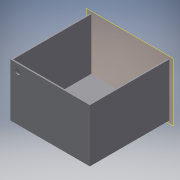
# Autodesk Inventor part: fixação chave geral
Saved by Autodesk Inventor 2019 (Build 230136000, 136)
## iProperties
Created: 2020-05-29
Part Number: fixação chave geral
Material: Generic
Document SubType Name: Modeling
Designer: luiza
Density: 1 g/cm^3
Appearance: Default
Author: luiza
Autodesk Inventor part; units mm, degrees
ref_plane "Work Plane1" through (0.1672, 0, 0) normal (0, 0, 1) x (1, 0, 0)
sketch "Sketch1" plane through (0.1672, 0, 0) normal (0, 0, 1) x (1, 0, 0)
  line L0 (-45.1672, 29.25) -> (44.8328, 29.25) projected
  line L1 (-45.1672, 29.25) -> (-45.1672, -30.75) projected
  line L2 (-45.1672, -30.75) -> (44.8328, -30.75) projected
  line L3 (44.8328, -30.75) -> (44.8328, 29.25) projected
  circle A0 centre (-37.1672, -22.75) radius 3 projected
  line L4 (44.8328, -30.75) -> (-45.1672, -30.75)
  line L5 (-45.1672, -30.75) -> (-45.1672, -29.25)
  line L6 (-45.1672, -29.25) -> (44.8328, -29.25)
  line L7 (44.8328, -29.25) -> (44.8328, -30.75)
  point P0 (-0.1672, 0)
  dimension "d0" = 1.5
  constraints: 8 end point, 2 parallel, 1 horizontal, 1 perpendicular, 1 point on line
  measures "d0" distance between parallel lines of L4 L6
ref_plane "Work Plane2" through (-45.2602, 13.6363, 90) normal (0, 0, 1) x (1, 0, 0)
extrude "Extrusion1" add sketch "Sketch1" along normal up to surface (90 mm away) contours L6 L3 L2 L1
sketch "Sketch2" plane through (-45, -29.25, 0) normal (0, 1, 0) x (1, 0, 0)
  line L0 (90, 0) -> (90, -90) projected
  line L1 (0, 0) -> (0, -90) projected
  line L2 (90, -90) -> (0, -90)
  line L3 (0, -90) -> (0, -88.5)
  line L4 (0, -88.5) -> (90, -88.5)
  line L5 (90, -88.5) -> (90, -90)
  point P0 (45, 0)
  dimension "d3" = 1.5
  constraints: 8 end point, 2 parallel, 1 horizontal, 1 perpendicular, 1 point on line
  measures "d3" distance between parallel lines of L2 L4
ref_plane "Work Plane3" through (-81.5561, 29.25, -36.5561) normal (0, -1, 0) x (1, 0, 0)
extrude "Extrusion2" add sketch "Sketch2" along normal up to surface (58.5 mm away)
sketch "Sketch4" plane through (-45, -29.25, 0) normal (0, 1, 0) x (1, 0, 0)
  line L0 (90, 0) -> (90, -88.5) projected
  line L1 (90, 0) -> (0, 0) projected
  line L2 (90, -88.5) -> (88.5, -88.5)
  line L3 (88.5, -88.5) -> (88.5, 0)
  line L4 (88.5, 0) -> (90, 0)
  line L5 (90, 0) -> (90, -88.5)
  line L6 (0, 0) -> (0, -88.5) projected
  line L7 (0, -88.5) -> (1.5, -88.5)
  line L8 (1.5, -88.5) -> (1.5, 0)
  line L9 (1.5, 0) -> (0, 0)
  line L10 (0, 0) -> (0, -88.5)
  point P0 (45, 0)
  dimension "d7" = 1.5
  dimension "d8" = 1.5
  constraints: 16 end point, 4 parallel, 2 horizontal, 2 perpendicular, 2 point on line
  measures "d7" distance between parallel lines of L0 L3
  measures "d8" distance between parallel lines of L6 L8
ref_plane "Work Plane4" through (-81.5561, 29.25, -36.5561) normal (0, -1, 0) x (1, 0, 0)
extrude "Extrusion3" add sketch "Sketch4" along normal up to surface (58.5 mm away)
sketch "Sketch5" plane through (-45, -30.75, 0) normal (0, -1, 0) x (1, 0, 0)
  circle A0 centre (82, 8) radius 3 projected
  point P0 (45, 0)
extrude "Extrusion4" cut sketch "Sketch5" against normal up to next
sketch "Sketch6" plane through (-45, -30.75, 90) normal (0, 0, 1) x (1, 0, 0)
  circle A0 centre (8, 52) radius 3 projected
  point P0 (45, 30.75)
extrude "Extrusion5" cut sketch "Sketch6" against normal up to next
body "Solid1"
